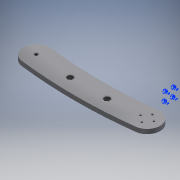
# Autodesk Inventor part: Arm 12X
Saved by Autodesk Inventor 2017 (Build 210142000, 142)
## iProperties
Created: 2016-03-22
Part Number: Arm 12X
Material: Generic
Document SubType Name: Modeling
Designer: alist
Density: 1 g/cm^3
Appearance: Default
Author: alist
Autodesk Inventor part; units mm, degrees
ref_plane "YZ Plane" through (0, 0, 0) normal (1, 0, 0) x (0, 1, 0)
ref_plane "XZ Plane" through (0, 0, 0) normal (0, 1, 0) x (-1, 0, 0)
ref_plane "XY Plane" through (0, 0, 0) normal (0, 0, 1) x (1, 0, 0)
sketch "Sketch1" plane through (0, 0, 0) normal (0, 0, 1) x (1, 0, 0)
  arc A0 (-74.2, 0) -> (74.2, 0) centre (0, 603.0231) ccw construction
  arc A1 (-76.3128, -17.1705) -> (76.3128, -17.1705) centre (0, 603.0231) ccw
  arc A2 (-72.0872, 17.1705) -> (72.0872, 17.1705) centre (0, 603.0231) ccw
  arc A3 (-72.0872, 17.1705) -> (-76.3128, -17.1705) centre (-74.2, 0) ccw
  arc A4 (76.3128, -17.1705) -> (72.0872, 17.1705) centre (74.2, 0) ccw
  line L0 (-159.9202, 0) -> (186.0645, 0) construction
  line L1 (0, 827.4607) -> (0, -503.7998) construction
  line L2 (74.2, 0) -> (74.2, 0) construction
  line L3 (74.2, 0) -> (91.3705, 2.1128) construction
  line L4 (74.2, 0) -> (72.0872, 17.1705) construction
  circle A5 centre (74.2, 0) radius 8 construction
  circle A6 centre (73.223, 7.9401) radius 1.15
  circle A7 centre (66.2599, -0.977) radius 1.15
  circle A8 centre (75.177, -7.9401) radius 1.15
  circle A9 centre (82.1401, 0.977) radius 1.15
  circle A10 centre (-74.2, 0) radius 2.15
  circle A11 centre (-24.7333, -4.0442) radius 2.15
  circle A12 centre (24.7333, -4.0442) radius 2.15
  point P0 (0, 0)
  dimension "d3" = 16
  dimension "d0" = 148.4
  dimension "d1" = 34.6
  dimension "d2" = 603.0231
  dimension "d4" = 2.3
  dimension "d7" = 360
  dimension "d9" = 49.4667
  dimension "d10" = 24.7333
  dimension "d11" = 4.3
  dimension "d12" = 4.3
  dimension "d13" = 4.3
  dimension "d46" = 7.015
  constraints: 14 point on circle, 12 centre point, 10 end point, 6 point on line, 6 tangent, 5 coincident, 1 horizontal, 1 perpendicular, 1 vertical, 12 other
  measures "d0" distance of A0.start L2.start
  measures "d1" diameter of A4
  measures "d2" distance from line of A0.centre L0
  measures "d4" diameter of A6
  measures "d9" distance of point (24.733, -4.044) point (-24.733, -4.044)
  measures "d10" horizontal distance of point (24.733, -4.044) point (0, 0)
  measures "d11" diameter of A10
  measures "d12" diameter of A11
  measures "d13" diameter of A12
  measures "d46" angle of L3 L0
extrude "Extrusion1" add sketch "Sketch1" along normal blind 6 contours A3 A2 A4 A1 | A6 | A7 | A8 | A9
sketch "Sketch2" plane through (0, 0, 6) normal (0, 0, 1) x (1, 0, 0)
  circle A0 centre (-24.7333, -4.0442) radius 2.15 projected
  line L0 (-21.0756, -6.0794) -> (-24.667, -8.2295)
  line L1 (-24.667, -8.2295) -> (-28.3247, -6.1943)
  line L2 (-28.3247, -6.1943) -> (-28.3911, -2.0091)
  line L3 (-28.3911, -2.0091) -> (-24.7997, 0.141)
  line L4 (-24.7997, 0.141) -> (-21.142, -1.8941)
  line L5 (-21.142, -1.8941) -> (-21.0756, -6.0794)
  circle A1 centre (24.7333, -4.0442) radius 2.15 projected
  line L6 (21.2567, -6.3753) -> (20.9762, -2.199)
  line L7 (20.9762, -2.199) -> (24.4529, 0.1321)
  line L8 (24.4529, 0.1321) -> (28.2099, -1.7132)
  line L9 (28.2099, -1.7132) -> (28.4904, -5.8895)
  line L10 (28.4904, -5.8895) -> (25.0138, -8.2206)
  line L11 (25.0138, -8.2206) -> (21.2567, -6.3753)
  point P0 (0, 0)
  dimension "d16" = 7.25
  dimension "d22" = 7.25
  constraints: 24 end point, 2 coincident, 26 other
  measures "d16" distance between parallel lines of L4 L1
  measures "d22" distance between parallel lines of L10 L7
extrude "Extrusion2" cut sketch "Sketch2" against normal blind 2
chamfer "Chamfer1" distance 2 angle 45 2 edges at (-26.8833, -4.0442, 4) (22.5833, -4.0442, 4)
sketch "Sketch4" plane through (0, 0, 0) normal (0, 0, -1) x (-1, 0, 0)
  line L0 (-73.223, 7.9401) -> (-75.177, -7.9401) construction
  circle A0 centre (-74.2, 0) radius 8 construction
  line L1 (-66.2, 0) -> (-95.5949, 0) construction
  line L2 (-66.2, 0) -> (0, 0) construction
  circle A1 centre (-75.177, -7.9401) radius 1.15 construction
  circle A2 centre (-66.2599, -0.977) radius 1.15 construction
  circle A3 centre (-73.223, 7.9401) radius 1.15 construction
  circle A4 centre (-82.1401, 0.977) radius 1.15 construction
  dimension "d28" = 82.985
  dimension "d29" = 16
  dimension "d30" = 2.3
  dimension "d31" = 74.2
  dimension "d34" = 360
  constraints: 6 end point, 5 centre point, 2 coincident, 2 horizontal, 2 midpoint, 2 point on circle, 2 point on line, 9 other
  measures "d28" angle of L1 L0
  measures "d29" diameter of A0
  measures "d30" diameter of A1
  measures "d31" distance of L2.end A0.centre
hole "Hole1" at (75.177, -7.9401, 0) at (82.1401, 0.977, 0) at (73.223, 7.9401, 0) at (66.2599, -0.977, 0) direction (0, 0, 1) diameter 2.3 end through all counterbore diameter 4.5 counterbore depth 2
chamfer "Chamfer2" distance 1.1 angle 45 4 edges at (75.177, -9.0901, 2) (82.1401, -0.173, 2) (66.2599, -2.127, 2) (73.223, 6.7901, 2)
equation "\"d9\" = 0.333333 * d0"
equation "\"d10\" = 0.5 * d9"
equation "\"d22\" = d16"
body "Solid1"
